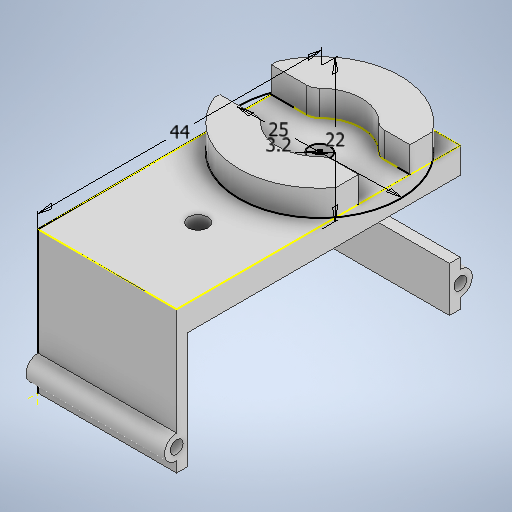
# Autodesk Inventor part: Gripper3overhead
Saved by Autodesk Inventor 2025.2 (Build 292293000, 293)
## iProperties
Created: 2025-03-30
Part Number: Gripper3overhead
Material: Generic
Document SubType Name: Modeling
Designer: m_kni
Density: 1 g/cm^3
Appearance: Default
Author: m_kni
## iProperties of the stored document Gripper3overhead_3DPrint.ipt
Created: 2025-04-02
Part Number: Gripper3overhead_3DPrint
Material: Generic
Document SubType Name: Modeling
Designer: m_kni
Density: 1 g/cm^3
Appearance: Default
Author: m_kni
Autodesk Inventor part; units mm, degrees
ref_plane "YZ Plane" through (0, 0, 0) normal (1, 0, 0) x (0, 1, 0)
ref_plane "XZ Plane" through (0, 0, 0) normal (0, 1, 0) x (-1, 0, 0)
ref_plane "XY Plane" through (0, 0, 0) normal (0, 0, 1) x (1, 0, 0)
sketch "Sketch1" plane through (0, 0, 0) normal (0, 1, 0) x (-1, 0, 0)
  line L0 (-10, -20.125) -> (10, -20.125)
  line L1 (10, -20.125) -> (10, 20.125)
  line L2 (10, 20.125) -> (-10, 20.125)
  line L3 (-10, 20.125) -> (-10, -20.125)
  line L4 (-10, -20.125) -> (10, 20.125) construction
  line L5 (10, -20.125) -> (-10, 20.125) construction
  line L6 (-11.5, -22) -> (11.5, -22)
  line L7 (11.5, -22) -> (11.5, 22)
  line L8 (11.5, 22) -> (-11.5, 22)
  line L9 (-11.5, 22) -> (-11.5, -22)
  line L10 (-11.5, -22) -> (11.5, 22) construction
  line L11 (11.5, -22) -> (-11.5, 22) construction
  line L12 (-10, 20.125) -> (-10, 22)
  line L13 (-10, -20.125) -> (-10, -22)
  point P0 (0, 0)
  dimension "d0" = 20
  dimension "d1" = 40.25
  dimension "d2" = 23
  dimension "d3" = 44
  constraints: 28 end point, 4 midpoint, 4 parallel, 4 point on line, 2 horizontal, 2 perpendicular
  measures "d0" distance of L2.end L1.end
  measures "d1" distance of L1.end L0.end
  measures "d2" distance of L8.end L7.end
  measures "d3" distance of L7.end L6.end
extrude "Extrusion1" add sketch "Sketch1" along normal blind 7 contours L0 L1 L2 L12 L8 L7 L6 L13
sketch "Sketch2" plane through (-11.5, 0, -22) normal (-1, 0, 0) x (0, 0, 1)
  line L0 (44, 0) -> (0, 0)
  line L1 (0, 0) -> (0, 22)
  line L2 (0, 22) -> (44, 22)
  line L3 (44, 22) -> (44, 0)
  point P0 (22, 0)
  dimension "d6" = 44
  dimension "d7" = 22
  constraints: 8 end point, 2 parallel, 1 horizontal, 1 perpendicular
  measures "d6" distance of L1.end L2.end
  measures "d7" distance of L0.end L1.end
sketch "Sketch3" plane through (0, 7, 0) normal (0, 1, 0) x (1, 0, 0)
  line L0 (-10, -20.125) -> (-10, 20.125) projected
  line L1 (-10, 20.125) -> (10, 20.125) projected
  line L2 (10, 20.125) -> (10, 22) projected
  line L3 (10, 22) -> (-11.5, 22) projected
  line L4 (-11.5, 22) -> (-11.5, -22) projected
  line L5 (-11.5, -22) -> (10, -22) projected
  line L6 (10, -22) -> (10, -20.125) projected
  line L7 (10, -20.125) -> (-10, -20.125) projected
  line L8 (-10, 20.125) -> (-10, 22)
  point P0 (0, 0)
  constraints: 2 end point, 1 perpendicular, 1 point on line
extrude "Extrusion2" add sketch "Sketch3" along normal blind 11 contours L7 L6 L5 L4 L3 L8 L0
sketch "Sketch4" plane through (0, 18, 0) normal (0, 1, 0) x (1, 0, 0)
  line L0 (10, -22) -> (10, -20.125) projected
  line L1 (-10, 22) -> (-11.5, 22) projected
  line L2 (10, -22) -> (-11.5, -22)
  line L3 (-11.5, -22) -> (-11.5, 22)
  line L4 (-11.5, 22) -> (10, 22)
  line L5 (10, 22) -> (10, -22)
  point P0 (0, 0)
  constraints: 8 end point, 2 parallel, 1 horizontal, 1 perpendicular
extrude "Extrusion3" add sketch "Sketch4" along normal blind 4
sketch "Sketch5" plane through (0, 22, 0) normal (0, 1, 0) x (1, 0, 0)
  line L0 (10, 20.125) -> (10, 22) projected
  line L1 (10, 22) -> (-11.5, 22) projected
  line L2 (10, 22) -> (-11.5, 22)
  circle A0 centre (0, 10.2) radius 6.5
  circle A1 centre (0, 10.2) radius 9
  line L3 (0, 10.2) -> (-11.5, 10.2)
  line L4 (-11.5, 22) -> (-11.5, -22) projected
  line L5 (0, 10.2) -> (0, 14.2)
  line L6 (0, 14.2) -> (-11.5, 14.2)
  line L7 (0, 10.2) -> (0, 6.2)
  line L8 (0, 6.2) -> (-11.5, 6.2)
  line L9 (0, 6.2) -> (10, 6.2)
  line L10 (0, 14.2) -> (10, 14.2)
  line L11 (10, -22) -> (10, 22) projected
  line L12 (-11.5, -22) -> (10, -22) projected
  line L13 (10, -22) -> (10, 22) projected
  line L14 (10, 22) -> (-11.5, 22) projected
  line L15 (-11.5, 22) -> (-11.5, -22) projected
  point P0 (0, 0)
  point P1 (0, 22)
  point P2 (5.1235, 14.2)
  point P3 (8.0623, 14.2)
  point P4 (-8.0623, 14.2)
  point P5 (-5.1235, 14.2)
  point P6 (8.0623, 6.2)
  point P7 (5.1235, 6.2)
  point P8 (-5.1235, 6.2)
  point P9 (-8.0623, 6.2)
  dimension "d12" = 11.8
  dimension "d13" = 13
  dimension "d14" = 18
  dimension "d15" = 4
  dimension "d16" = 4
  constraints: 16 end point, 7 point on line, 3 perpendicular, 2 centre point, 2 coincident, 2 horizontal, 1 collinear
  measures "d12" distance from line of L1 point (0, 10.2)
  measures "d13" diameter of A0
  measures "d14" diameter of A1
  measures "d15" distance of L3.start L5.end
  measures "d16" distance of L3.start L7.end
extrude "Extrusion4" add sketch "Sketch5" along normal blind 4 contours L10 A0 L6 A1 | A1 L8 A0 L9
fillet "Fillet1" radius 2 4 edges at (-5.1235, 24, -14.2) (5.1235, 24, -14.2) (-5.1235, 24, -6.2) (5.1235, 24, -6.2)
sketch "Sketch6" plane through (0, 22, 0) normal (0, 1, 0) x (1, 0, 0)
  line L0 (8.0623, 14.2) -> (6.0208, 14.2) projected
  arc A0 (4.6041, 14.7882) -> (6.0208, 14.2) centre (6.0208, 16.2) ccw projected
  arc A1 (4.6041, 14.7882) -> (-4.6041, 14.7882) centre (0, 10.2) ccw projected
  arc A2 (-6.0208, 14.2) -> (-4.6041, 14.7882) centre (-6.0208, 16.2) ccw projected
  line L1 (-6.0208, 14.2) -> (-8.0623, 14.2) projected
  arc A3 (8.0623, 14.2) -> (-8.0623, 14.2) centre (0, 10.2) ccw projected
  line L2 (6.0208, 6.2) -> (8.0623, 6.2) projected
  arc A4 (-8.0623, 6.2) -> (8.0623, 6.2) centre (0, 10.2) ccw projected
  line L3 (-8.0623, 6.2) -> (-6.0208, 6.2) projected
  arc A5 (-4.6041, 5.6118) -> (-6.0208, 6.2) centre (-6.0208, 4.2) ccw projected
  arc A6 (-4.6041, 5.6118) -> (4.6041, 5.6118) centre (0, 10.2) ccw projected
  arc A7 (6.0208, 6.2) -> (4.6041, 5.6118) centre (6.0208, 4.2) ccw projected
  line L4 (-11.5, -22) -> (10, -22) projected
  line L5 (10, -22) -> (10, 22) projected
  line L6 (10, 22) -> (-11.5, 22) projected
  line L7 (-11.5, 22) -> (-11.5, -22) projected
  arc A8 (6.0208, 6.2) -> (4.6041, 5.6118) centre (6.0208, 4.2) ccw projected
  arc A9 (-4.6041, 5.6118) -> (4.6041, 5.6118) centre (0, 10.2) ccw projected
  arc A10 (-4.6041, 5.6118) -> (-6.0208, 6.2) centre (-6.0208, 4.2) ccw projected
  line L8 (-6.0208, 6.2) -> (-8.0623, 6.2) projected
  arc A11 (-8.0623, 6.2) -> (8.0623, 6.2) centre (0, 10.2) ccw projected
  line L9 (8.0623, 6.2) -> (6.0208, 6.2) projected
  arc A12 (4.6041, 14.7882) -> (6.0208, 14.2) centre (6.0208, 16.2) ccw projected
  line L10 (6.0208, 14.2) -> (8.0623, 14.2) projected
  arc A13 (8.0623, 14.2) -> (-8.0623, 14.2) centre (0, 10.2) ccw projected
  line L11 (-8.0623, 14.2) -> (-6.0208, 14.2) projected
  arc A14 (-6.0208, 14.2) -> (-4.6041, 14.7882) centre (-6.0208, 16.2) ccw projected
  arc A15 (4.6041, 14.7882) -> (-4.6041, 14.7882) centre (0, 10.2) ccw projected
  line L12 (-8.0623, 6.2) -> (-11.5, 6.2)
  line L13 (-8.0623, 14.2) -> (-11.5, 14.2)
  line L14 (-11.5, 22) -> (-11.5, -22) projected
  line L15 (8.0623, 6.2) -> (10, 6.2)
  line L16 (8.0623, 14.2) -> (10, 14.2)
  circle A16 centre (0, 10.2) radius 12.5
  circle A17 centre (0, 10.2) radius 1.6
  point P0 (0, 0)
  point P1 (-11.5, 5.301)
  point P2 (10, 2.7)
  point P3 (10, 17.7)
  point P4 (-11.5, 15.099)
  dimension "d20" = 25
  dimension "d21" = 3.2
  constraints: 8 end point, 6 point on line, 2 centre point, 2 coincident, 1 horizontal, 1 perpendicular
  measures "d20" diameter of A16
  measures "d21" diameter of A17
extrude "Extrusion5" add sketch "Sketch6" along normal up to surface (4 mm away) contours A3 L13 L7 A16 L6 L5 L16 | L5 A16 L7 L12 A4 L15 | L6 A16
extrude "Extrusion6" cut sketch "Sketch6" against normal blind 10 contours A17
sketch "Sketch7" plane through (10, 0, -20.125) normal (1, 0, 0) x (0, 0, -1)
  line L0 (0, 0) -> (1.875, 0) projected
  line L1 (1.875, 0) -> (1.875, 7) projected
  line L2 (0, 7) -> (1.875, 7) projected
  line L3 (0, 0) -> (0, 7) projected
  line L4 (-42.125, 0) -> (-40.25, 0) projected
  line L5 (-40.25, 0) -> (-40.25, 18) projected
  line L6 (-40.25, 18) -> (1.875, 18) projected
  line L7 (1.875, 18) -> (1.875, 22) projected
  line L8 (-2.425, 22) -> (1.875, 22) projected
  line L9 (-2.425, 22) -> (-2.425, 26) projected
  line L10 (-2.425, 26) -> (-5.925, 26) projected
  line L11 (-5.925, 22) -> (-5.925, 26) projected
  line L12 (-13.925, 22) -> (-5.925, 22) projected
  line L13 (-13.925, 22) -> (-13.925, 26) projected
  line L14 (-13.925, 26) -> (-17.425, 26) projected
  line L15 (-17.425, 22) -> (-17.425, 26) projected
  line L16 (-42.125, 22) -> (-17.425, 22) projected
  line L17 (-42.125, 0) -> (-42.125, 22) projected
  line L18 (1.875, 0) -> (1.875, 7) projected
  circle A0 centre (1.875, 3.5) radius 1.875
  line L19 (-42.125, 0) -> (-42.125, 22) projected
  circle A1 centre (-42.125, 3.5) radius 1.875
  point P0 (-20.125, 0)
  point P1 (-42.125, 5.375)
  point P2 (-42.125, 1.625)
  point P3 (1.875, 5.375)
  point P4 (1.875, 1.625)
  dimension "d26" = 3.75
  dimension "d27" = 3.75
  constraints: 2 centre point, 1 midpoint, 1 point on line
  measures "d26" diameter of A0
  measures "d27" diameter of A1
extrude "Extrusion7" add sketch "Sketch7" against normal up to surface (21.5 mm away) contours L1 A0 | A1 L17 picked at (2.2647, 3.9886) picked at (-43.0085, 3.7216)
sketch "Sketch8" plane through (10, 0, -20.125) normal (1, 0, 0) x (0, 0, -1)
  line L0 (0, 0) -> (1.875, 0) projected
  line L1 (1.875, 0) -> (1.875, 1.625) projected
  arc A0 (1.875, 1.625) -> (1.875, 5.375) centre (1.875, 3.5) ccw projected
  line L2 (1.875, 5.375) -> (1.875, 7) projected
  line L3 (0, 7) -> (1.875, 7) projected
  line L4 (0, 0) -> (0, 7) projected
  line L5 (-42.125, 0) -> (-40.25, 0) projected
  line L6 (-40.25, 0) -> (-40.25, 18) projected
  line L7 (-40.25, 18) -> (1.875, 18) projected
  line L8 (1.875, 18) -> (1.875, 22) projected
  line L9 (-2.425, 22) -> (1.875, 22) projected
  line L10 (-2.425, 22) -> (-2.425, 26) projected
  line L11 (-2.425, 26) -> (-5.925, 26) projected
  line L12 (-5.925, 22) -> (-5.925, 26) projected
  line L13 (-13.925, 22) -> (-5.925, 22) projected
  line L14 (-13.925, 22) -> (-13.925, 26) projected
  line L15 (-13.925, 26) -> (-17.425, 26) projected
  line L16 (-17.425, 22) -> (-17.425, 26) projected
  line L17 (-42.125, 22) -> (-17.425, 22) projected
  line L18 (-42.125, 5.375) -> (-42.125, 22) projected
  arc A1 (-42.125, 5.375) -> (-42.125, 1.625) centre (-42.125, 3.5) ccw projected
  line L19 (-42.125, 0) -> (-42.125, 1.625) projected
  circle A2 centre (-42.125, 3.5) radius 1
  circle A3 centre (1.875, 3.5) radius 1
  point P0 (-20.125, 0)
  dimension "d30" = 2
  dimension "d31" = 2
  constraints: 2 centre point, 2 coincident
  measures "d30" diameter of A2
  measures "d31" diameter of A3
extrude "Extrusion8" cut sketch "Sketch8" against normal blind 6 contours A2 | A3
sketch "Sketch9" plane through (10, 0, 22) normal (1, 0, 0) x (0, 0, -1)
  line L0 (1.875, 0) -> (1.875, 18) projected
  line L1 (44, 0) -> (0, 0) projected
  line L2 (1.875, 18) -> (1.675, 18)
  line L3 (1.675, 18) -> (1.675, 0)
  line L4 (1.675, 0) -> (1.875, 0)
  line L5 (1.875, 0) -> (1.875, 18)
  line L6 (42.125, 0) -> (42.125, 7) projected
  line L7 (42.125, 0) -> (44, 0) projected
  line L8 (42.125, 7) -> (42.325, 7)
  line L9 (42.325, 7) -> (42.325, 0)
  line L10 (42.325, 0) -> (42.125, 0)
  line L11 (42.125, 0) -> (42.125, 7)
  point P0 (22, 0)
  dimension "d34" = 0.2
  dimension "d35" = 0.2
  constraints: 16 end point, 4 parallel, 2 horizontal, 2 perpendicular, 2 point on line
  measures "d34" distance of L4.end L3.end
  measures "d35" distance of L9.end L10.end
extrude "Extrusion9" cut sketch "Sketch9" against normal up to surface (20 mm away)
sketch "Sketch10" plane through (-10, 7, -22) normal (1, 0, 0) x (0, 0, -1)
  line L0 (-42.325, -7) -> (-1.675, -7) projected
  line L1 (-1.675, 0) -> (-1.675, -7) projected
  line L2 (0, 0) -> (-1.675, 0) projected
  line L3 (0, 0) -> (0, 11) projected
  line L4 (-42.325, 11) -> (0, 11) projected
  line L5 (-42.325, -7) -> (-42.325, 11) projected
  line L6 (0, 0) -> (-1.675, 0)
  line L7 (-1.675, 0) -> (-1.675, 11)
  line L8 (-1.675, 11) -> (0, 11)
  line L9 (0, 11) -> (0, 0)
  point P0 (-22, -7)
  constraints: 8 end point, 2 parallel, 1 horizontal, 1 perpendicular, 1 point on line
extrude "Extrusion10" add sketch "Sketch10" along normal blind 5 contours L7 L4 L3 L2
sketch "Sketch11" plane through (0, 18, 0) normal (0, -1, 0) x (1, 0, 0)
  circle A0 centre (0, 8.6768) radius 1.5
  point P0 (0, 0)
  dimension "d40" = 3
  constraints: 1 centre point
  measures "d40" diameter of A0
extrude "Extrusion11" cut sketch "Sketch11" against normal blind 5
body "Solid1"
